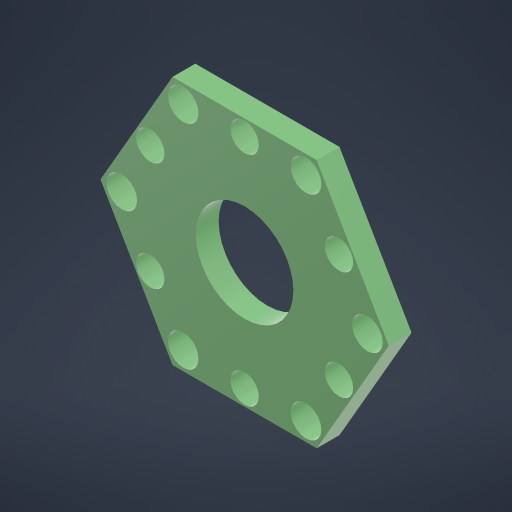
# Autodesk Inventor part: 90d Spacer
Saved by Autodesk Inventor 2024.2 (Build 282272000, 272)
## iProperties
Created: 2022-10-16
Part Number: 90d Spacer
Material: Generic
Document SubType Name: Modeling
Designer: Jason
Density: 1 g/cm^3
Appearance: Smooth - Dark Forest Green
Author: Jason
Autodesk Inventor part; units mm, degrees
ref_plane "YZ Plane" through (0, 0, 0) normal (1, 0, 0) x (0, 1, 0)
ref_plane "XZ Plane" through (0, 0, 0) normal (0, 1, 0) x (-1, 0, 0)
ref_plane "XY Plane" through (0, 0, 0) normal (0, 0, 1) x (1, 0, 0)
sketch "Sketch1" plane through (0, 0, 0) normal (0, 0, 1) x (1, 0, 0)
  line L0 (-9.3881, 16.2606) -> (9.3868, 16.2606)
  line L1 (18.7092, 0.25) -> (18.7092, 0.25)
  line L2 (18.7762, 0) -> (9.3868, 16.2606)
  line L3 (18.7762, 0) -> (9.3868, -16.2606)
  line L4 (-9.3881, -16.2606) -> (9.3868, -16.2606)
  line L5 (-18.7762, 0) -> (-9.3881, -16.2606)
  line L6 (-18.7762, 0) -> (-9.3881, 16.2606)
  circle A0 centre (16, 0) radius 2
  circle A1 centre (8, 13.8564) radius 2
  circle A2 centre (-8, 13.8564) radius 2
  circle A3 centre (-16, 0) radius 2
  circle A4 centre (8, -13.8564) radius 2
  circle A5 centre (-8, -13.8564) radius 2
  circle A6 centre (0, 0) radius 6.35
  circle A7 centre (-0.0003, -14.1904) radius 1.8542
  circle A8 centre (0.001, 14.1866) radius 1.8542
  circle A9 centre (12.2905, 7.0829) radius 1.8542
  circle A10 centre (12.2905, -7.0852) radius 1.8542
  circle A11 centre (-12.2865, -7.0924) radius 1.8542
  circle A12 centre (-12.2865, 7.0829) radius 1.8542
  dimension "d3" = 12.7
  dimension "d4" = 3.7084
  dimension "d5" = 3.7084
  dimension "d6" = 3.7084
  dimension "d7" = 3.7084
  dimension "d8" = 3.7084
  dimension "d9" = 3.7084
  constraints: 14 end point, 13 centre point, 2 horizontal
  measures "d3" diameter of A6
  measures "d4" diameter of A7
  measures "d5" diameter of A8
  measures "d6" diameter of A9
  measures "d7" diameter of A10
  measures "d8" diameter of A11
  measures "d9" diameter of A12
extrude "Extrusion1" add sketch "Sketch1" along normal blind 2.9718
